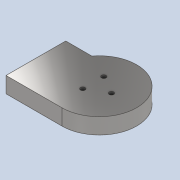
# Autodesk Inventor part: FFS080YS102U6
Saved by Autodesk Inventor 2022 (Build 260153000, 153)
## iProperties
Created: 2023-06-19
Part Number: FFS080YS102U6
Material: ステンレス鋼
Document SubType Name: Modeling
Designer: 81805
Density: 8 g/cm^3
Appearance: 半つや出し
Author: 81805
Autodesk Inventor part; units mm, degrees
ref_plane "YZ Plane" through (0, 0, 0) normal (1, 0, 0) x (0, 1, 0)
ref_plane "XZ Plane" through (0, 0, 0) normal (0, 1, 0) x (-1, 0, 0)
ref_plane "XY Plane" through (0, 0, 0) normal (0, 0, 1) x (1, 0, 0)
sketch "スケッチ1" plane through (0, 0, 0) normal (0, 0, 1) x (1, 0, 0)
  arc A0 (40, 0) -> (-24, -32) centre (0, 0) ccw
  line L0 (40, 0) -> (-24, 0)
  line L1 (-24, -32) -> (-24, -60)
  line L2 (-24, -60) -> (40, -60)
  line L3 (40, -60) -> (40, 0)
  circle A1 centre (0, 0) radius 13
  point P0 (-24, -32)
  point P1 (0, 13)
  point P2 (-11.2583, -6.5)
  point P3 (11.2583, -6.5)
  dimension "d12" = 26
  dimension "d0" = 80
  dimension "d1" = 0
  dimension "d2" = 64
  dimension "d3" = 60
  dimension "d15" = 360
  dimension "d17" = 0
  constraints: 8 end point, 2 coincident, 2 parallel, 2 point on circle, 1 centre point, 1 horizontal, 1 perpendicular, 1 vertical alignment, 6 other
  measures "d0" diameter of A0
  measures "d1" distance from line of L0 point (0, 0)
  measures "d2" distance of L1.end L2.end
  measures "d3" distance from line of A0.centre L2
  measures "d17" horizontal distance of point (0, 0) point (0, 13)
extrude "押し出し1" add sketch "スケッチ1" against normal blind 17 contours L3 L2 L1 A0 | A1 L0 | L0 A1
hole "穴1" at (0, 13, 0) at (-11.2583, -6.5, 0) at (11.2583, -6.5, 0) direction (0, 0, -1) diameter 4.917 depth 10 tip angle 118 thread size "M6x1" class "6H" standard "ISO Metric profile"
